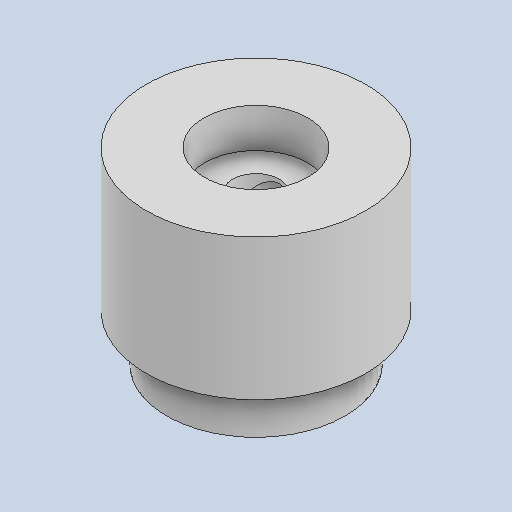
# Autodesk Inventor part: vial
Saved by Autodesk Inventor 2025 (Build 290162010, 162A)
## iProperties
Created: 2023-05-02
Part Number: vial
Material: Generic
Document SubType Name: Modeling
Designer: dinesh
Density: 1 g/cm^3
Appearance: Default
Author: dinesh
Autodesk Inventor part; units mm, degrees
ref_plane "YZ Plane" through (0, 0, 0) normal (1, 0, 0) x (0, 1, 0)
ref_plane "XZ Plane" through (0, 0, 0) normal (0, 1, 0) x (-1, 0, 0)
ref_plane "XY Plane" through (0, 0, 0) normal (0, 0, 1) x (1, 0, 0)
sketch "Sketch1" plane through (0, 0, 0) normal (0, 0, 1) x (1, 0, 0)
  line L0 (3, 12) -> (14, 12)
  line L1 (14, 12) -> (14, 0)
  line L2 (3, 2) -> (3, 12)
  line L3 (0, 19.5472) -> (0, -22.4151)
  line L4 (14, 0) -> (13, 0) construction
  line L5 (13, 0) -> (13, -6)
  line L6 (13, -6) -> (14, -6)
  line L7 (14, -6) -> (14, 0)
  line L8 (11.4, 0) -> (10.4, 0) construction
  line L9 (10.4, 0) -> (10.4, -6) construction
  line L10 (10.4, -6) -> (11.4, -6) construction
  line L11 (11.4, -6) -> (11.4, 0)
  line L12 (11.4, -6) -> (11.4, -12)
  line L13 (11.4, -12) -> (11.3, -12)
  line L14 (11.3, -12) -> (10.4892, -6.5945)
  arc A0 (3, 2) -> (4.4967, 0.0644) centre (5, 2) ccw
  line L15 (13, 0) -> (11.4, 0)
  line L16 (10.4, 0) -> (5, 0)
  line L17 (-20.0393, 0) -> (13, 0) construction
  line L18 (14, 0) -> (24.5476, 0) construction
  line L19 (5.48, -0.5334) -> (9.9979, -5.5532)
  arc A1 (10.4892, -6.5945) -> (9.9979, -5.5532) centre (8.5113, -6.8911) ccw
  arc A2 (5.48, -0.5334) -> (4.4967, 0.0644) centre (3.9934, -1.8713) ccw
  point P0 (0, 0)
  point P1 (10.4, 0)
  point P2 (10.5, -6)
  dimension "d0" = 6
  dimension "d2" = 1
  dimension "d4" = 1
  dimension "d5" = 6
  dimension "d6" = 1.6
  dimension "d7" = 26
  dimension "d9" = 6
  dimension "d10" = 0.1
  dimension "d11" = 2
  dimension "d12" = 12
  dimension "d14" = 6
  dimension "d41" = 2
  dimension "d42" = 2
  constraints: 40 end point, 8 point on line, 7 parallel, 7 point on circle, 6 horizontal, 6 tangent, 4 collinear, 4 perpendicular, 3 centre point, 3 vertical, 1 equal radius, 4 other
  measures "d0" diameter of L2 L3
  measures "d2" distance between parallel lines of L5 L7
  measures "d4" distance between parallel lines of L11 L9
  measures "d5" distance between parallel lines of L10 L8
  measures "d6" distance between parallel lines of L5 L11
  measures "d7" diameter of L5 L3
  measures "d9" distance of L10.end L12.end
  measures "d10" distance of L12.end L13.end
  measures "d11" radius of A0
  measures "d12" distance between parallel lines of L16 L0
  measures "d14" distance between parallel lines of L6 L4
  measures "d41" radius of A1
  measures "d42" radius of A2
revolve "Revolution1" add sketch "Sketch1" angle 360 about axis through (0, 19.5472, 0) along (0, -1, 0)
sketch "Sketch2" plane through (0, 0, 0) normal (0, 0, 1) x (1, 0, 0)
  line L0 (-3, 12) -> (3, 12) projected
  line L1 (0, 12) -> (0, 0) construction
  line L2 (-3, 2) -> (3, 2) construction
  circle A0 centre (0, 3.5) radius 3
  line L3 (-13, 0) -> (13, 0) construction
  point P0 (2.5981, 2)
  point P1 (-2.5981, 2)
  dimension "d16" = 6
  dimension "d43" = 3.5
  constraints: 2 end point, 1 centre point, 1 midpoint, 1 perpendicular, 1 point on line
  measures "d16" diameter of A0
  measures "d43" distance from line of L3 A0.centre
extrude "Extrusion1" cut sketch "Sketch2" along normal blind 3 and the other way blind 19.5
sketch "Sketch4" plane through (0, 12, 0) normal (0, 1, 0) x (1, 0, 0)
  circle A0 centre (0, 0) radius 6.6
  dimension "d38" = 13.2
  constraints: 1 centre point, 1 coincident
  measures "d38" diameter of A0
extrude "Extrusion3" cut sketch "Sketch4" against normal blind 5
sketch "Sketch3" plane through (0, 12, 0) normal (0, 1, 0) x (1, 0, 0)
  circle A0 centre (-5.25, 0) radius 0.45
  line L0 (0, 0) -> (-14, 0) construction
  circle A1 centre (0, 0) radius 14 construction
  circle A2 centre (-7.5, 0) radius 0.45
  circle A3 centre (0, 0) radius 3 construction
  arc A4 (-2.5981, 1.5) -> (-2.5981, -1.5) centre (0, 0) ccw construction
  circle A5 centre (-6.4952, -3.75) radius 0.45
  circle A6 centre (-4.5466, -2.625) radius 0.45
  circle A7 centre (-3.75, -6.4952) radius 0.45
  circle A8 centre (-2.625, -4.5466) radius 0.45
  circle A9 centre (0, -7.5) radius 0.45
  circle A10 centre (0, -5.25) radius 0.45
  circle A11 centre (3.75, -6.4952) radius 0.45
  circle A12 centre (2.625, -4.5466) radius 0.45
  circle A13 centre (6.4952, -3.75) radius 0.45
  circle A14 centre (4.5466, -2.625) radius 0.45
  circle A15 centre (7.5, 0) radius 0.45
  circle A16 centre (5.25, 0) radius 0.45
  circle A17 centre (6.4952, 3.75) radius 0.45
  circle A18 centre (4.5466, 2.625) radius 0.45
  circle A19 centre (3.75, 6.4952) radius 0.45
  circle A20 centre (2.625, 4.5466) radius 0.45
  circle A21 centre (0, 7.5) radius 0.45
  circle A22 centre (0, 5.25) radius 0.45
  circle A23 centre (-3.75, 6.4952) radius 0.45
  circle A24 centre (-2.625, 4.5466) radius 0.45
  circle A25 centre (-6.4952, 3.75) radius 0.45
  circle A26 centre (-4.5466, 2.625) radius 0.45
  point P0 (-3, 0)
  point P1 (-3, 0)
  dimension "d22" = 0.9
  dimension "d24" = 0.9
  dimension "d30" = 2.25
  dimension "d31" = 2.25
  dimension "d34" = 360
  constraints: 24 centre point, 3 point on line, 2 end point, 2 point on circle, 1 horizontal, 1 horizontal alignment, 50 other
  measures "d22" diameter of A0
  measures "d24" diameter of A2
  measures "d30" distance of A2.centre A0.centre
  measures "d31" distance of point (-3, 0) A0.centre
equation "\"d0\" = t_D"
equation "\"d2\" = w_th"
equation "\"d4\" = w_th"
equation "\"d5\" = w_l"
equation "\"d6\" = lv_th"
equation "\"d7\" = lv_OD"
equation "\"d9\" = w_l"
equation "\"d10\" = tol"
equation "\"d11\" = fillet_D"
equation "\"d12\" = top_th_f"
equation "\"d14\" = w_l"
equation "\"d41\" = fillet_D"
equation "\"d42\" = fillet_D"
equation "\"d16\" = t_D"
equation "\"d43\" = 0.5 * w_th + 0.5 * t_D"
equation "\"d18\" = 0.5 * t_D"
equation "\"d19\" = 0.75 * lv_OD"
equation "\"d38\" = cn_D"
equation "\"d39\" = cn_h"
equation "\"d22\" = h_D"
equation "\"d24\" = h_D"
equation "\"d30\" = h_s"
equation "\"d31\" = h_s"
equation "\"tol\" = 0.1"
equation "\"fillet_D\" = 2"
equation "\"w_th\" = 1"
equation "\"w_l\" = 6"
equation "\"t_D\" = 6"
equation "\"t_D_f\" = t_D + w_th"
equation "\"top_th_f\" = t_D_f + cn_h"
equation "\"cn_h\" = 5"
equation "\"lv_OD\" = 26"
equation "\"lv_th\" = 1.6"
equation "\"d3\" = w_l"
equation "\"d8\" = top_th_f"
equation "\"top_th\" = t_D + w_th"
equation "\"sv_OD\" = 13"
equation "\"sv_th\" = 1.5"
equation "\"b_OD\" = 44"
equation "\"b_th\" = 1.5"
equation "\"b_ID\" = 36.5"
equation "\"b_rim_h\" = 5"
equation "\"h_s\" = 2.25"
equation "\"h_D\" = 0.9"
equation "\"d25\" = 2 * d26"
equation "\"v_h_D\" = 7.5"
equation "\"v_h_off\" = 0.5 * cn_D + 0.5 * v_h_D"
equation "\"cn_D\" = 13.2"
equation "\"d26\" = 0.1"
body "Solid1"
